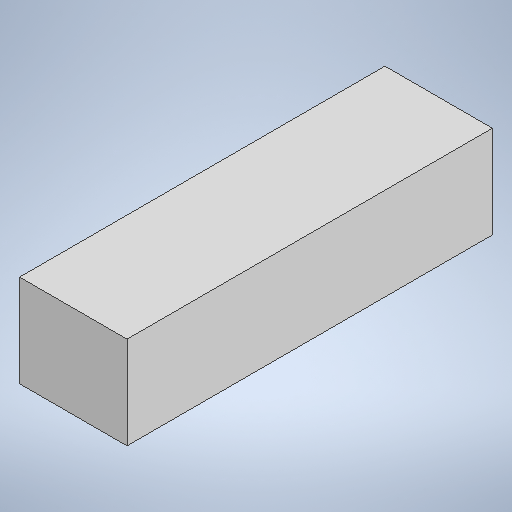
# Autodesk Inventor part: Battery
Saved by Autodesk Inventor 2025 (Build 290162000, 162)
## iProperties
Created: 2024-08-30
Part Number: Battery
Material: Generic
Document SubType Name: Modeling
Designer: Cupri
Density: 1 g/cm^3
Appearance: Default
Author: Cupri
Autodesk Inventor part; units mm, degrees
ref_plane "YZ Plane" through (0, 0, 0) normal (1, 0, 0) x (0, 1, 0)
ref_plane "XZ Plane" through (0, 0, 0) normal (0, 1, 0) x (-1, 0, 0)
ref_plane "XY Plane" through (0, 0, 0) normal (0, 0, 1) x (1, 0, 0)
sketch "Sketch1" plane through (0, 0, 0) normal (0, 0, 1) x (1, 0, 0)
  line L0 (-25, -21.5) -> (25, -21.5)
  line L1 (25, -21.5) -> (25, 21.5)
  line L2 (25, 21.5) -> (-25, 21.5)
  line L3 (-25, 21.5) -> (-25, -21.5)
  line L4 (-25, -21.5) -> (25, 21.5) construction
  line L5 (25, -21.5) -> (-25, 21.5) construction
  point P0 (0, 0)
  dimension "d0" = 50
  dimension "d1" = 43
  constraints: 12 end point, 2 midpoint, 2 parallel, 1 horizontal, 1 perpendicular
  measures "d0" distance of L1.end L2.end
  measures "d1" distance of L0.end L1.end
extrude "Extrusion1" add sketch "Sketch1" along normal blind 170
body "Solid1"
